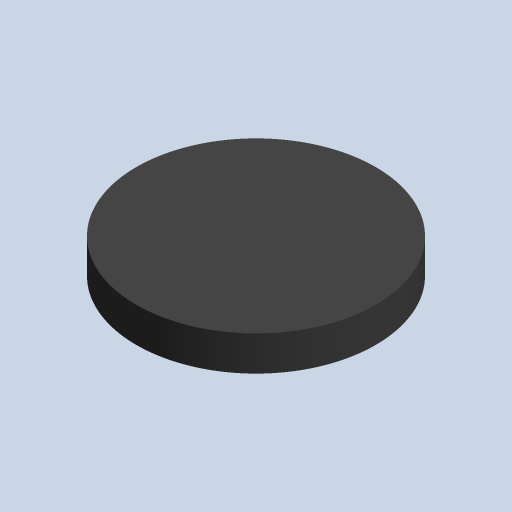
# Autodesk Inventor part: seal
Saved by Autodesk Inventor 2024 (Build 280153000, 153)
## iProperties
Part Number: seal
Material: Generic
Document SubType Name: Modeling
Designer: newic
Appearance: Default
Author: newic
Autodesk Inventor part; units mm, degrees
ref_plane "YZ Plane" through (0, 0, 0) normal (1, 0, 0) x (0, 1, 0)
ref_plane "XZ Plane" through (0, 0, 0) normal (0, 1, 0) x (-1, 0, 0)
ref_plane "XY Plane" through (0, 0, 0) normal (0, 0, 1) x (1, 0, 0)
sketch "Sketch1" plane through (0, 0, 0) normal (0, 1, 0) x (-1, 0, 0)
  line L0 (0, 0) -> (76.2002, 0) construction
  line L1 (76.2002, 0) -> (76.2002, -76.2002) construction
  line L2 (76.2002, -76.2002) -> (0, -76.2002) construction
  line L3 (0, -76.2002) -> (0, 0) construction
  circle A0 centre (38.1001, -38.1001) radius 21.8573
  circle A1 centre (38.1001, -38.1001) radius 20.8567
  line L4 (40.6618, -37.2458) -> (41.1876, -36.742)
  line L5 (41.1876, -36.742) -> (41.1876, -32.9593)
  spline S0 degree 4 poles (41.1876, -32.9593) (41.2926, -32.7172) (41.0043, -32.7956) (41.135, -32.4515) (40.8057, -32.605) knots 0 0 0 0 0 1 1 1 1 1
  line L6 (40.8057, -32.605) -> (40.0393, -32.605)
  arc A2 (40.0393, -31.6655) -> (40.0393, -32.605) centre (40.17, -32.1352) ccw
  line L7 (40.0393, -31.6655) -> (44.4894, -31.6655)
  arc A3 (44.4894, -32.605) -> (44.4894, -31.6655) centre (44.3665, -32.1352) ccw
  arc A4 (43.5252, -32.605) -> (43.1544, -32.9593) centre (43.4942, -32.9437) ccw
  line L8 (43.5252, -32.605) -> (44.4894, -32.605)
  line L9 (43.1544, -32.9593) -> (43.1544, -43.4953)
  line L10 (43.1544, -43.4953) -> (43.1877, -43.6584) construction
  line L11 (43.1877, -43.6584) -> (43.3031, -43.8163) construction
  line L12 (43.3031, -43.8163) -> (43.4033, -43.8706) construction
  line L13 (43.4033, -43.8706) -> (43.573, -43.9418) construction
  line L14 (43.573, -43.9418) -> (43.84, -44.0167) construction
  line L15 (43.84, -44.0167) -> (44.112, -44.0167) construction
  line L16 (44.112, -44.0167) -> (44.5627, -44.11) construction
  line L17 (44.5627, -44.11) -> (44.6715, -44.1722) construction
  line L18 (44.6715, -44.1722) -> (44.9163, -44.3198) construction
  line L19 (44.9163, -44.3198) -> (45.0154, -44.4232) construction
  line L20 (45.0154, -44.4232) -> (45.0834, -44.5452) construction
  line L21 (45.0834, -44.5452) -> (45.0834, -44.6618) construction
  line L22 (45.0834, -44.6618) -> (45.1145, -44.7939) construction
  line L23 (45.1145, -44.7939) -> (44.9878, -44.9153) construction
  line L24 (44.9878, -44.9153) -> (44.7842, -45.0076) construction
  line L25 (44.7842, -45.0076) -> (44.6482, -45.0076) construction
  spline S1 degree 4 poles (43.1544, -43.4953) (43.1877, -43.6584) (43.3031, -43.8163) (43.4033, -43.8706) (43.573, -43.9418) (43.84, -44.0167) (44.112, -44.0167) (44.5627, -44.11) (44.6715, -44.1722) (44.9163, -44.3198) (45.0154, -44.4232) (45.0834, -44.5452) (45.0834, -44.6618) (45.1145, -44.7939) (44.9878, -44.9153) (44.7842, -45.0076) (44.6482, -45.0076) knots 1 1 1 1 1 2 3 4 5 6 7 8 9 10 11 12 13 14 14 14 14 14
  arc A5 (44.6482, -45.0076) -> (39.9953, -45.0076) centre (42.3218, -57.2669) ccw
  line L26 (39.9953, -45.0076) -> (39.6196, -45.0402) construction
  line L27 (39.6196, -45.0402) -> (39.4833, -44.9615) construction
  line L28 (39.4833, -44.9615) -> (39.3855, -44.9153) construction
  line L29 (39.3855, -44.9153) -> (39.2941, -44.7888) construction
  line L30 (39.2941, -44.7888) -> (39.2941, -44.6035) construction
  line L31 (39.2941, -44.6035) -> (39.3481, -44.504) construction
  line L32 (39.3481, -44.504) -> (39.4207, -44.3715) construction
  line L33 (39.4207, -44.3715) -> (39.6288, -44.2164) construction
  line L34 (39.6288, -44.2164) -> (39.9032, -44.1411) construction
  line L35 (39.9032, -44.1411) -> (40.2033, -44.0797) construction
  line L36 (40.2033, -44.0797) -> (40.4675, -44.0634) construction
  line L37 (40.4675, -44.0634) -> (40.7103, -44.0167) construction
  line L38 (40.7103, -44.0167) -> (40.902, -43.9418) construction
  line L39 (40.902, -43.9418) -> (41.1242, -43.7775) construction
  line L40 (41.1242, -43.7775) -> (41.2453, -43.71) construction
  line L41 (41.2453, -43.71) -> (41.2975, -43.5237) construction
  spline S2 degree 4 poles (39.9953, -45.0076) (39.6196, -45.0402) (39.4833, -44.9615) (39.3855, -44.9153) (39.2941, -44.7888) (39.2941, -44.6035) (39.3481, -44.504) (39.4207, -44.3715) (39.6288, -44.2164) (39.9032, -44.1411) (40.2033, -44.0797) (40.4675, -44.0634) (40.7103, -44.0167) (40.902, -43.9418) (41.1242, -43.7775) (41.2453, -43.71) (41.2975, -43.5237) knots 1 1 1 1 1 2 3 4 5 6 7 8 9 10 11 12 13 14 14 14 14 14
  line L42 (41.2975, -43.5237) -> (41.2975, -40.0842)
  line L43 (41.2975, -40.0842) -> (40.7103, -39.4498)
  line L44 (40.7103, -39.4498) -> (34.7202, -39.4498)
  line L45 (40.6618, -37.2458) -> (34.7686, -37.2458)
  line L46 (34.7686, -37.2458) -> (34.2429, -36.742)
  line L47 (34.2429, -36.742) -> (34.2429, -32.9593)
  spline S3 degree 4 poles (34.2429, -32.9593) (34.1682, -32.7875) (34.3486, -32.6326) (34.3667, -32.6001) (34.6248, -32.605) knots 0 0 0 0 0 1 1 1 1 1
  line L48 (34.6248, -32.605) -> (35.3912, -32.605)
  arc A6 (35.3912, -32.605) -> (35.3912, -31.6655) centre (35.2605, -32.1352) ccw
  line L49 (35.3912, -31.6655) -> (30.941, -31.6655)
  arc A7 (30.941, -31.6655) -> (30.941, -32.605) centre (31.064, -32.1352) ccw
  arc A8 (32.2761, -32.9593) -> (31.9052, -32.605) centre (31.9363, -32.9437) ccw
  line L50 (31.9052, -32.605) -> (30.941, -32.605)
  line L51 (32.2761, -32.9593) -> (32.2761, -43.4953)
  line L52 (32.2761, -43.4953) -> (32.2427, -43.6584) construction
  line L53 (32.2427, -43.6584) -> (32.1273, -43.8163) construction
  line L54 (32.1273, -43.8163) -> (32.0272, -43.8706) construction
  line L55 (32.0272, -43.8706) -> (31.8575, -43.9418) construction
  line L56 (31.8575, -43.9418) -> (31.5905, -44.0167) construction
  line L57 (31.5905, -44.0167) -> (31.3185, -44.0167) construction
  line L58 (31.3185, -44.0167) -> (30.8677, -44.11) construction
  line L59 (30.8677, -44.11) -> (30.7589, -44.1722) construction
  line L60 (30.7589, -44.1722) -> (30.5141, -44.3198) construction
  line L61 (30.5141, -44.3198) -> (30.415, -44.4232) construction
  line L62 (30.415, -44.4232) -> (30.347, -44.5452) construction
  line L63 (30.347, -44.5452) -> (30.347, -44.6618) construction
  line L64 (30.347, -44.6618) -> (30.316, -44.7939) construction
  line L65 (30.316, -44.7939) -> (30.4426, -44.9153) construction
  line L66 (30.4426, -44.9153) -> (30.6462, -45.0076) construction
  line L67 (30.6462, -45.0076) -> (30.7822, -45.0076) construction
  spline S4 degree 4 poles (32.2761, -43.4953) (32.2427, -43.6584) (32.1273, -43.8163) (32.0272, -43.8706) (31.8575, -43.9418) (31.5905, -44.0167) (31.3185, -44.0167) (30.8677, -44.11) (30.7589, -44.1722) (30.5141, -44.3198) (30.415, -44.4232) (30.347, -44.5452) (30.347, -44.6618) (30.316, -44.7939) (30.4426, -44.9153) (30.6462, -45.0076) (30.7822, -45.0076) knots 1 1 1 1 1 2 3 4 5 6 7 8 9 10 11 12 13 14 14 14 14 14
  arc A9 (35.4351, -45.0076) -> (30.7822, -45.0076) centre (33.1087, -57.2669) ccw
  line L68 (35.4351, -45.0076) -> (35.8108, -45.0402) construction
  line L69 (35.8108, -45.0402) -> (35.9472, -44.9615) construction
  line L70 (35.9472, -44.9615) -> (36.0449, -44.9153) construction
  line L71 (36.0449, -44.9153) -> (36.1363, -44.7888) construction
  line L72 (36.1363, -44.7888) -> (36.1363, -44.6035) construction
  line L73 (36.1363, -44.6035) -> (36.0824, -44.504) construction
  line L74 (36.0824, -44.504) -> (36.0098, -44.3715) construction
  line L75 (36.0098, -44.3715) -> (35.8017, -44.2164) construction
  line L76 (35.8017, -44.2164) -> (35.5273, -44.1411) construction
  line L77 (35.5273, -44.1411) -> (35.2272, -44.0797) construction
  line L78 (35.2272, -44.0797) -> (34.963, -44.0634) construction
  line L79 (34.963, -44.0634) -> (34.7202, -44.0167) construction
  line L80 (34.7202, -44.0167) -> (34.5284, -43.9418) construction
  line L81 (34.5284, -43.9418) -> (34.3063, -43.7775) construction
  line L82 (34.3063, -43.7775) -> (34.1852, -43.71) construction
  line L83 (34.1852, -43.71) -> (34.1329, -43.5237) construction
  spline S5 degree 4 poles (35.4351, -45.0076) (35.8108, -45.0402) (35.9472, -44.9615) (36.0449, -44.9153) (36.1363, -44.7888) (36.1363, -44.6035) (36.0824, -44.504) (36.0098, -44.3715) (35.8017, -44.2164) (35.5273, -44.1411) (35.2272, -44.0797) (34.963, -44.0634) (34.7202, -44.0167) (34.5284, -43.9418) (34.3063, -43.7775) (34.1852, -43.71) (34.1329, -43.5237) knots 1 1 1 1 1 2 3 4 5 6 7 8 9 10 11 12 13 14 14 14 14 14
  line L84 (34.1329, -43.5237) -> (34.1329, -40.0842)
  line L85 (34.1329, -40.0842) -> (34.7202, -39.4498)
  line L86 (34.7202, -39.4498) -> (40.7103, -39.4498)
  line L87 (38.2912, -52.5831) -> (38.0672, -52.5831)
  line L88 (48.7025, -50.0158) -> (49.2279, -50.0158)
  line L89 (49.2279, -50.0158) -> (49.761, -50.4057)
  line L90 (49.761, -50.4057) -> (49.8872, -50.2845) construction
  line L91 (49.8872, -50.2845) -> (50.0462, -50.1321) construction
  line L92 (50.0462, -50.1321) -> (50.1401, -49.9591) construction
  line L93 (50.1401, -49.9591) -> (50.3738, -49.7351) construction
  line L94 (50.3738, -49.7351) -> (50.6671, -49.443) construction
  line L95 (50.6671, -49.443) -> (50.9264, -49.1944) construction
  line L96 (50.9264, -49.1944) -> (51.1372, -48.9924) construction
  line L97 (51.1372, -48.9924) -> (51.7205, -48.3816) construction
  line L98 (51.7205, -48.3816) -> (52.1066, -47.8535) construction
  line L99 (52.1066, -47.8535) -> (52.4867, -47.4569) construction
  line L100 (52.4867, -47.4569) -> (52.8214, -46.9579) construction
  line L101 (52.8214, -46.9579) -> (53.2913, -46.4144) construction
  line L102 (53.2913, -46.4144) -> (53.7244, -45.822) construction
  line L103 (53.7244, -45.822) -> (53.8819, -45.6067) construction
  line L104 (53.8819, -45.6067) -> (54.0234, -45.2698) construction
  line L105 (54.0234, -45.2698) -> (54.098, -45.1983) construction
  line L106 (54.098, -45.1983) -> (54.069, -45.1461) construction
  line L107 (54.069, -45.1461) -> (54.0322, -45.1077) construction
  line L108 (54.0322, -45.1077) -> (53.8711, -44.9534) construction
  line L109 (53.8711, -44.9534) -> (53.6017, -44.6962) construction
  line L110 (53.6017, -44.6962) -> (53.2876, -44.11) construction
  line L111 (53.2876, -44.11) -> (52.7307, -43.3484) construction
  line L112 (52.7307, -43.3484) -> (52.267, -42.5166) construction
  line L113 (52.267, -42.5166) -> (51.2177, -40.6344) construction
  line L114 (51.2177, -40.6344) -> (50.2882, -38.5878) construction
  line L115 (50.2882, -38.5878) -> (49.761, -37.085) construction
  line L116 (49.761, -37.085) -> (49.1388, -35.28) construction
  line L117 (49.1388, -35.28) -> (48.4341, -32.6978) construction
  line L118 (48.4341, -32.6978) -> (48.4341, -32.3678) construction
  line L119 (48.4341, -32.3678) -> (48.2809, -31.6655) construction
  line L120 (48.2809, -31.6655) -> (48.2661, -31.5479) construction
  spline S6 degree 4 poles (49.761, -50.4057) (49.8872, -50.2845) (50.0462, -50.1321) (50.1401, -49.9591) (50.3738, -49.7351) (50.6671, -49.443) (50.9264, -49.1944) (51.1372, -48.9924) (51.7205, -48.3816) (52.1066, -47.8535) (52.4867, -47.4569) (52.8214, -46.9579) (53.2913, -46.4144) (53.7244, -45.822) (53.8819, -45.6067) (54.0234, -45.2698) (54.098, -45.1983) (54.069, -45.1461) (54.0322, -45.1077) (53.8711, -44.9534) (53.6017, -44.6962) (53.2876, -44.11) (52.7307, -43.3484) (52.267, -42.5166) (51.2177, -40.6344) (50.2882, -38.5878) (49.761, -37.085) (49.1388, -35.28) (48.4341, -32.6978) (48.4341, -32.3678) (48.2809, -31.6655) (48.2661, -31.5479) knots 1 1 1 1 1 2 3 4 5 6 7 8 9 10 11 12 13 14 15 16 17 18 19 20 21 22 23 24 25 26 27 28 29 29 29 29 29
  line L121 (48.2661, -31.5479) -> (48.2274, -31.2403) construction
  line L122 (48.2274, -31.2403) -> (48.2541, -30.9327) construction
  line L123 (48.2541, -30.9327) -> (48.2541, -30.7642) construction
  line L124 (48.2541, -30.7642) -> (48.3417, -30.5558) construction
  line L125 (48.3417, -30.5558) -> (48.3952, -30.5045) construction
  line L126 (48.3952, -30.5045) -> (48.5589, -30.5384) construction
  line L127 (48.5589, -30.5384) -> (48.7025, -30.6473) construction
  line L128 (48.7025, -30.6473) -> (48.8728, -30.8478) construction
  line L129 (48.8728, -30.8478) -> (49.1688, -31.1565) construction
  line L130 (49.1688, -31.1565) -> (49.5553, -31.6852) construction
  line L131 (49.5553, -31.6852) -> (49.8872, -32.0507) construction
  line L132 (49.8872, -32.0507) -> (50.2882, -32.3413) construction
  line L133 (50.2882, -32.3413) -> (50.6084, -32.4076) construction
  line L134 (50.6084, -32.4076) -> (50.7152, -32.3052) construction
  line L135 (50.7152, -32.3052) -> (50.9957, -32.2478) construction
  line L136 (50.9957, -32.2478) -> (51.3083, -31.9482) construction
  line L137 (51.3083, -31.9482) -> (51.4714, -31.7252) construction
  line L138 (51.4714, -31.7252) -> (51.7423, -31.4649) construction
  line L139 (51.7423, -31.4649) -> (51.9587, -31.4195) construction
  line L140 (51.9587, -31.4195) -> (52.142, -31.2439) construction
  line L141 (52.142, -31.2439) -> (52.267, -31.1341) construction
  line L142 (52.267, -31.1341) -> (52.1937, -31.0543) construction
  line L143 (52.1937, -31.0543) -> (52.1066, -30.9669) construction
  line L144 (52.1066, -30.9669) -> (51.9585, -30.9254) construction
  line L145 (51.9585, -30.9254) -> (51.6761, -30.867) construction
  line L146 (51.6761, -30.867) -> (51.5091, -30.6926) construction
  line L147 (51.5091, -30.6926) -> (51.2639, -30.5134) construction
  line L148 (51.2639, -30.5134) -> (51.1401, -30.3836) construction
  line L149 (51.1401, -30.3836) -> (51.0087, -30.2039) construction
  line L150 (51.0087, -30.2039) -> (51.0087, -29.9872) construction
  line L151 (51.0087, -29.9872) -> (51.1613, -29.775) construction
  line L152 (51.1613, -29.775) -> (51.5939, -29.3746) construction
  line L153 (51.5939, -29.3746) -> (51.9135, -29.0787) construction
  line L154 (51.9135, -29.0787) -> (52.1836, -28.8286) construction
  line L155 (52.1836, -28.8286) -> (52.3342, -28.4702) construction
  line L156 (52.3342, -28.4702) -> (52.6833, -27.9927) construction
  line L157 (52.6833, -27.9927) -> (52.9107, -27.5734) construction
  line L158 (52.9107, -27.5734) -> (53.0092, -27.2183) construction
  line L159 (53.0092, -27.2183) -> (52.7307, -26.5536) construction
  line L160 (52.7307, -26.5536) -> (52.4989, -26.1497) construction
  line L161 (52.4989, -26.1497) -> (52.1641, -25.9049) construction
  line L162 (52.1641, -25.9049) -> (51.1372, -25.108) construction
  line L163 (51.1372, -25.108) -> (50.3531, -24.635) construction
  line L164 (50.3531, -24.635) -> (49.721, -24.211) construction
  line L165 (49.721, -24.211) -> (49.1894, -23.9238) construction
  line L166 (49.1894, -23.9238) -> (48.8873, -23.6086) construction
  line L167 (48.8873, -23.6086) -> (48.2185, -23.1196) construction
  line L168 (48.2185, -23.1196) -> (47.9551, -22.7594) construction
  line L169 (47.9551, -22.7594) -> (47.6777, -22.4563) construction
  line L170 (47.6777, -22.4563) -> (47.3154, -22.3042) construction
  line L171 (47.3154, -22.3042) -> (47.0473, -22.1916) construction
  line L172 (47.0473, -22.1916) -> (46.6874, -22.1916) construction
  line L173 (46.6874, -22.1916) -> (46.317, -22.2339) construction
  line L174 (46.317, -22.2339) -> (45.9234, -22.3551) construction
  line L175 (45.9234, -22.3551) -> (45.2614, -22.5181) construction
  line L176 (45.2614, -22.5181) -> (44.803, -22.7218) construction
  line L177 (44.803, -22.7218) -> (44.304, -22.9323) construction
  line L178 (44.304, -22.9323) -> (42.7641, -23.6271) construction
  spline S7 degree 4 poles (48.2661, -31.5479) (48.2274, -31.2403) (48.2541, -30.9327) (48.2541, -30.7642) (48.3417, -30.5558) (48.3952, -30.5045) (48.5589, -30.5384) (48.7025, -30.6473) (48.8728, -30.8478) (49.1688, -31.1565) (49.5553, -31.6852) (49.8872, -32.0507) (50.2882, -32.3413) (50.6084, -32.4076) (50.7152, -32.3052) (50.9957, -32.2478) (51.3083, -31.9482) (51.4714, -31.7252) (51.7423, -31.4649) (51.9587, -31.4195) (52.142, -31.2439) (52.267, -31.1341) (52.1937, -31.0543) (52.1066, -30.9669) (51.9585, -30.9254) (51.6761, -30.867) (51.5091, -30.6926) (51.2639, -30.5134) (51.1401, -30.3836) (51.0087, -30.2039) (51.0087, -29.9872) (51.1613, -29.775) (51.5939, -29.3746) (51.9135, -29.0787) (52.1836, -28.8286) (52.3342, -28.4702) (52.6833, -27.9927) (52.9107, -27.5734) (53.0092, -27.2183) (52.7307, -26.5536) (52.4989, -26.1497) (52.1641, -25.9049) (51.1372, -25.108) (50.3531, -24.635) (49.721, -24.211) (49.1894, -23.9238) (48.8873, -23.6086) (48.2185, -23.1196) (47.9551, -22.7594) (47.6777, -22.4563) (47.3154, -22.3042) (47.0473, -22.1916) (46.6874, -22.1916) (46.317, -22.2339) (45.9234, -22.3551) (45.2614, -22.5181) (44.803, -22.7218) (44.304, -22.9323) (42.7641, -23.6271) (42.1419, -23.8519) (41.7933, -23.9841) (41.6423, -24.0391) knots 1 1 1 1 1 2 3 4 5 6 7 8 9 10 11 12 13 14 15 16 17 18 19 20 21 22 23 24 25 26 27 28 29 30 31 32 33 34 35 36 37 38 39 40 41 42 43 44 45 46 47 48 49 50 51 52 53 54 55 56 57 58 58.816263 58.816263 58.816263 58.816263 58.816263
  line L179 (39.2968, -24.3991) -> (40.7554, -24.3991)
  line L180 (40.7554, -24.3991) -> (41.6423, -24.0391)
  line L181 (42.7641, -23.6271) -> (42.1419, -23.8519) construction
  line L182 (42.1419, -23.8519) -> (41.7933, -23.9841) construction
  line L183 (41.7933, -23.9841) -> (41.6423, -24.0391) construction
  line L184 (39.2968, -24.3991) -> (39.2433, -24.4111) construction
  line L185 (39.2433, -24.4111) -> (39.1663, -24.4723) construction
  line L186 (39.1663, -24.4723) -> (39.1175, -24.5601) construction
  line L187 (39.1175, -24.5601) -> (39.0699, -24.7134) construction
  line L188 (39.0699, -24.7134) -> (39.0012, -25.0007) construction
  line L189 (39.0012, -25.0007) -> (38.7576, -25.3192) construction
  line L190 (38.7576, -25.3192) -> (38.4704, -25.6314) construction
  line L191 (38.4704, -25.6314) -> (38.1769, -25.9186) construction
  line L192 (38.1769, -25.9186) -> (38.0838, -25.973) construction
  spline S8 degree 4 poles (39.2968, -24.3991) (39.2433, -24.4111) (39.1663, -24.4723) (39.1175, -24.5601) (39.0699, -24.7134) (39.0012, -25.0007) (38.7576, -25.3192) (38.4704, -25.6314) (38.1769, -25.9186) (38.0838, -25.973) knots 1 1 1 1 1 2 3 4 5 6 7 7 7 7 7
  line L193 (38.0838, -25.973) -> (37.6286, -25.973)
  line L194 (37.8562, -25.973) -> (38.1001, -56.7349)
  arc A10 (38.1001, -56.7349) -> (38.5091, -56.4718) centre (38.0456, -56.2007) ccw
  arc A11 (38.6312, -56.0666) -> (38.5091, -56.4718) centre (39.5479, -56.5638) ccw
  arc A12 (39.0699, -55.3511) -> (38.6312, -56.0666) centre (40.3438, -56.6243) ccw
  arc A13 (39.7556, -54.7188) -> (39.0699, -55.3511) centre (41.8297, -57.6563) ccw
  arc A14 (43.3532, -53.0725) -> (39.7556, -54.7188) centre (46.6536, -65.0391) ccw
  arc A15 (43.3532, -53.0725) -> (46.2754, -51.8022) centre (38.528, -37.9773) ccw
  arc A16 (46.2754, -51.8022) -> (48.7025, -50.0158) centre (44.0006, -46.1692) ccw
  line L195 (27.3925, -50.1848) -> (26.8671, -50.1931)
  line L196 (26.8671, -50.1931) -> (26.3403, -50.5913)
  line L197 (26.3403, -50.5913) -> (26.2121, -50.4722) construction
  line L198 (26.2121, -50.4722) -> (26.0508, -50.3224) construction
  line L199 (26.0508, -50.3224) -> (25.9542, -50.1509) construction
  line L200 (25.9542, -50.1509) -> (25.7169, -49.9306) construction
  line L201 (25.7169, -49.9306) -> (25.4191, -49.6431) construction
  line L202 (25.4191, -49.6431) -> (25.1558, -49.3987) construction
  line L203 (25.1558, -49.3987) -> (24.9419, -49.2001) construction
  line L204 (24.9419, -49.2001) -> (24.349, -48.5986) construction
  line L205 (24.349, -48.5986) -> (23.9545, -48.0767) construction
  line L206 (23.9545, -48.0767) -> (23.5682, -47.6861) construction
  line L207 (23.5682, -47.6861) -> (23.2255, -47.1925) construction
  line L208 (23.2255, -47.1925) -> (22.7471, -46.6565) construction
  line L209 (22.7471, -46.6565) -> (22.3047, -46.0711) construction
  line L210 (22.3047, -46.0711) -> (22.1438, -45.8583) construction
  line L211 (22.1438, -45.8583) -> (21.997, -45.5237) construction
  line L212 (21.997, -45.5237) -> (21.9212, -45.4533) construction
  line L213 (21.9212, -45.4533) -> (21.9495, -45.4007) construction
  line L214 (21.9495, -45.4007) -> (21.9857, -45.3618) construction
  line L215 (21.9857, -45.3618) -> (22.1442, -45.2049) construction
  line L216 (22.1442, -45.2049) -> (22.4095, -44.9434) construction
  line L217 (22.4095, -44.9434) -> (22.7143, -44.3524) construction
  line L218 (22.7143, -44.3524) -> (23.259, -43.5821) construction
  line L219 (23.259, -43.5821) -> (23.7095, -42.743) construction
  line L220 (23.7095, -42.743) -> (24.7289, -40.8444) construction
  line L221 (24.7289, -40.8444) -> (25.6258, -38.7833) construction
  line L222 (25.6258, -38.7833) -> (26.1291, -37.2724) construction
  line L223 (26.1291, -37.2724) -> (26.7226, -35.4578) construction
  line L224 (26.7226, -35.4578) -> (27.3863, -32.8646) construction
  line L225 (27.3863, -32.8646) -> (27.381, -32.5347) construction
  line L226 (27.381, -32.5347) -> (27.5231, -31.8301) construction
  line L227 (27.5231, -31.8301) -> (27.536, -31.7122) construction
  spline S9 degree 4 poles (26.3403, -50.5913) (26.2121, -50.4722) (26.0508, -50.3224) (25.9542, -50.1509) (25.7169, -49.9306) (25.4191, -49.6431) (25.1558, -49.3987) (24.9419, -49.2001) (24.349, -48.5986) (23.9545, -48.0767) (23.5682, -47.6861) (23.2255, -47.1925) (22.7471, -46.6565) (22.3047, -46.0711) (22.1438, -45.8583) (21.997, -45.5237) (21.9212, -45.4533) (21.9495, -45.4007) (21.9857, -45.3618) (22.1442, -45.2049) (22.4095, -44.9434) (22.7143, -44.3524) (23.259, -43.5821) (23.7095, -42.743) (24.7289, -40.8444) (25.6258, -38.7833) (26.1291, -37.2724) (26.7226, -35.4578) (27.3863, -32.8646) (27.381, -32.5347) (27.5231, -31.8301) (27.536, -31.7122) knots 1 1 1 1 1 2 3 4 5 6 7 8 9 10 11 12 13 14 15 16 17 18 19 20 21 22 23 24 25 26 27 28 29 29 29 29 29
  line L228 (27.536, -31.7122) -> (27.5698, -31.4041) construction
  line L229 (27.5698, -31.4041) -> (27.5382, -31.0969) construction
  line L230 (27.5382, -31.0969) -> (27.5355, -30.9284) construction
  line L231 (27.5355, -30.9284) -> (27.4447, -30.7215) construction
  line L232 (27.4447, -30.7215) -> (27.3904, -30.671) construction
  line L233 (27.3904, -30.671) -> (27.2272, -30.7075) construction
  line L234 (27.2272, -30.7075) -> (27.0854, -30.8187) construction
  line L235 (27.0854, -30.8187) -> (26.9182, -31.0218) construction
  line L236 (26.9182, -31.0218) -> (26.6273, -31.3353) construction
  line L237 (26.6273, -31.3353) -> (26.2492, -31.8699) construction
  line L238 (26.2492, -31.8699) -> (25.9231, -32.2407) construction
  line L239 (25.9231, -32.2407) -> (25.5267, -32.5376) construction
  line L240 (25.5267, -32.5376) -> (25.2077, -32.609) construction
  line L241 (25.2077, -32.609) -> (25.0992, -32.5083) construction
  line L242 (25.0992, -32.5083) -> (24.8179, -32.4553) construction
  line L243 (24.8179, -32.4553) -> (24.5005, -32.1607) construction
  line L244 (24.5005, -32.1607) -> (24.3339, -31.9403) construction
  line L245 (24.3339, -31.9403) -> (24.0589, -31.6844) construction
  line L246 (24.0589, -31.6844) -> (23.8418, -31.6424) construction
  line L247 (23.8418, -31.6424) -> (23.6558, -31.4698) construction
  line L248 (23.6558, -31.4698) -> (23.529, -31.3619) construction
  line L249 (23.529, -31.3619) -> (23.6011, -31.281) construction
  line L250 (23.6011, -31.281) -> (23.6868, -31.1922) construction
  line L251 (23.6868, -31.1922) -> (23.8342, -31.1484) construction
  line L252 (23.8342, -31.1484) -> (24.1156, -31.0855) construction
  line L253 (24.1156, -31.0855) -> (24.2799, -30.9085) construction
  line L254 (24.2799, -30.9085) -> (24.5221, -30.7254) construction
  line L255 (24.5221, -30.7254) -> (24.6439, -30.5937) construction
  line L256 (24.6439, -30.5937) -> (24.7724, -30.4119) construction
  line L257 (24.7724, -30.4119) -> (24.769, -30.1953) construction
  line L258 (24.769, -30.1953) -> (24.6131, -29.9855) construction
  line L259 (24.6131, -29.9855) -> (24.1742, -29.5919) construction
  line L260 (24.1742, -29.5919) -> (23.8499, -29.3012) construction
  line L261 (23.8499, -29.3012) -> (23.5758, -29.0554) construction
  line L262 (23.5758, -29.0554) -> (23.4196, -28.6995) construction
  line L263 (23.4196, -28.6995) -> (23.0629, -28.2275) construction
  line L264 (23.0629, -28.2275) -> (22.8289, -27.8119) construction
  line L265 (22.8289, -27.8119) -> (22.7249, -27.4584) construction
  line L266 (22.7249, -27.4584) -> (22.9927, -26.7893) construction
  line L267 (22.9927, -26.7893) -> (23.2182, -26.3818) construction
  line L268 (23.2182, -26.3818) -> (23.549, -26.1318) construction
  line L269 (23.549, -26.1318) -> (24.5632, -25.3187) construction
  line L270 (24.5632, -25.3187) -> (25.3397, -24.8333) construction
  line L271 (25.3397, -24.8333) -> (25.9649, -24.3993) construction
  line L272 (25.9649, -24.3993) -> (26.492, -24.1038) construction
  line L273 (26.492, -24.1038) -> (26.789, -23.7838) construction
  line L274 (26.789, -23.7838) -> (27.45, -23.2843) construction
  line L275 (27.45, -23.2843) -> (27.7076, -22.9199) construction
  line L276 (27.7076, -22.9199) -> (27.9802, -22.6125) construction
  line L277 (27.9802, -22.6125) -> (28.34, -22.4546) construction
  line L278 (28.34, -22.4546) -> (28.6063, -22.3378) construction
  line L279 (28.6063, -22.3378) -> (28.9662, -22.3321) construction
  line L280 (28.9662, -22.3321) -> (29.3372, -22.3686) construction
  line L281 (29.3372, -22.3686) -> (29.7326, -22.4834) construction
  line L282 (29.7326, -22.4834) -> (30.3972, -22.6359) construction
  line L283 (30.3972, -22.6359) -> (30.8587, -22.8323) construction
  line L284 (30.8587, -22.8323) -> (31.361, -23.0349) construction
  line L285 (31.361, -23.0349) -> (32.9117, -23.7052) construction
  spline S10 degree 4 poles (27.536, -31.7122) (27.5698, -31.4041) (27.5382, -31.0969) (27.5355, -30.9284) (27.4447, -30.7215) (27.3904, -30.671) (27.2272, -30.7075) (27.0854, -30.8187) (26.9182, -31.0218) (26.6273, -31.3353) (26.2492, -31.8699) (25.9231, -32.2407) (25.5267, -32.5376) (25.2077, -32.609) (25.0992, -32.5083) (24.8179, -32.4553) (24.5005, -32.1607) (24.3339, -31.9403) (24.0589, -31.6844) (23.8418, -31.6424) (23.6558, -31.4698) (23.529, -31.3619) (23.6011, -31.281) (23.6868, -31.1922) (23.8342, -31.1484) (24.1156, -31.0855) (24.2799, -30.9085) (24.5221, -30.7254) (24.6439, -30.5937) (24.7724, -30.4119) (24.769, -30.1953) (24.6131, -29.9855) (24.1742, -29.5919) (23.8499, -29.3012) (23.5758, -29.0554) (23.4196, -28.6995) (23.0629, -28.2275) (22.8289, -27.8119) (22.7249, -27.4584) (22.9927, -26.7893) (23.2182, -26.3818) (23.549, -26.1318) (24.5632, -25.3187) (25.3397, -24.8333) (25.9649, -24.3993) (26.492, -24.1038) (26.789, -23.7838) (27.45, -23.2843) (27.7076, -22.9199) (27.9802, -22.6125) (28.34, -22.4546) (28.6063, -22.3378) (28.9662, -22.3321) (29.3372, -22.3686) (29.7326, -22.4834) (30.3972, -22.6359) (30.8587, -22.8323) (31.361, -23.0349) (32.9117, -23.7052) (33.5374, -23.9201) (33.8881, -24.0468) (34.0399, -24.0993) knots 1 1 1 1 1 2 3 4 5 6 7 8 9 10 11 12 13 14 15 16 17 18 19 20 21 22 23 24 25 26 27 28 29 30 31 32 33 34 35 36 37 38 39 40 41 42 43 44 45 46 47 48 49 50 51 52 53 54 55 56 57 58 58.816263 58.816263 58.816263 58.816263 58.816263
  line L286 (36.3908, -24.4221) -> (34.9324, -24.4452)
  line L287 (34.9324, -24.4452) -> (34.0399, -24.0993)
  line L288 (32.9117, -23.7052) -> (33.5374, -23.9201) construction
  line L289 (33.5374, -23.9201) -> (33.8881, -24.0468) construction
  line L290 (33.8881, -24.0468) -> (34.0399, -24.0993) construction
  line L291 (36.3908, -24.4221) -> (36.4445, -24.4333) construction
  line L292 (36.4445, -24.4333) -> (36.5225, -24.4932) construction
  line L293 (36.5225, -24.4932) -> (36.5727, -24.5802) construction
  line L294 (36.5727, -24.5802) -> (36.6227, -24.7328) construction
  line L295 (36.6227, -24.7328) -> (36.696, -25.019) construction
  line L296 (36.696, -25.019) -> (36.9445, -25.3335) construction
  line L297 (36.9445, -25.3335) -> (37.2367, -25.6412) construction
  line L298 (37.2367, -25.6412) -> (37.5347, -25.9237) construction
  line L299 (37.5347, -25.9237) -> (37.6287, -25.9766) construction
  spline S11 degree 4 poles (36.3908, -24.4221) (36.4445, -24.4333) (36.5225, -24.4932) (36.5727, -24.5802) (36.6227, -24.7328) (36.696, -25.019) (36.9445, -25.3335) (37.2367, -25.6412) (37.5347, -25.9237) (37.6287, -25.9766) knots 1 1 1 1 1 2 3 4 5 6 7 7 7 7 7
  line L300 (37.6287, -25.9766) -> (38.0837, -25.9694)
  arc A17 (29.8476, -51.9324) -> (32.7895, -53.1563) centre (37.3749, -37.9864) ccw
  arc A18 (27.3925, -50.1848) -> (29.8476, -51.9324) centre (32.0328, -46.2641) ccw
  arc A19 (36.1363, -54.4971) -> (32.7895, -53.1563) centre (28.5329, -68.6286) ccw
  arc A20 (37.5347, -55.923) -> (36.1363, -54.4971) centre (32.3957, -59.564) ccw
  arc A21 (37.5347, -55.923) -> (38.1001, -56.7349) centre (38.3931, -55.928) ccw
  line L301 (37.8765, -28.5293) -> (38.9353, -28.5293)
  spline S12 degree 4 poles (38.9353, -28.5293) (39.0734, -28.5153) (39.235, -28.4247) (39.7119, -27.9172) (40.0591, -27.4924) (40.3856, -27.2204) (40.628, -27.0204) (40.8114, -26.9226) (41.1862, -26.9437) (41.513, -26.9433) (41.6075, -26.8718) (42.1054, -26.7692) (42.4444, -26.5333) (42.9513, -26.4281) (43.3962, -26.1436) (43.8872, -26.1192) (44.318, -25.8883) (44.9007, -25.4806) (45.5398, -25.3135) (45.9229, -25.2078) (45.976, -25.0775) knots 0 0 0 0 0 0.112458 0.166879 0.220388 0.267174 0.311957 0.35453 0.394382 0.437668 0.482725 0.531671 0.587405 0.64421 0.700743 0.757907 0.816633 0.875573 1 1 1 1 1
  spline S13 degree 4 poles (45.976, -25.0775) (46.0524, -25.0518) (46.2811, -25.1254) (46.3903, -24.9958) (46.6702, -25.2353) (47.0934, -25.6298) (47.464, -26.0099) (48.1375, -26.4473) (48.7069, -26.8363) (48.9769, -27.0113) (49.2133, -27.1257) (49.3419, -27.2815) (49.4167, -27.3513) (49.417, -27.4775) (49.4428, -27.5915) (49.4153, -27.6867) (49.4243, -27.763) (49.3797, -27.8219) (49.2973, -27.8628) (49.0519, -27.8753) (48.2998, -27.8481) (47.8569, -27.8921) (47.342, -27.8307) (47.2381, -27.8825) knots 0 0 0 0 0 0.086112 0.127188 0.177084 0.240639 0.312756 0.380982 0.442012 0.491183 0.529078 0.56225 0.592572 0.620822 0.648025 0.672897 0.695594 0.720273 0.755564 0.802899 0.860568 1 1 1 1 1
  spline S14 degree 4 poles (47.2381, -27.8825) (46.8036, -28.0259) (47.051, -28.1864) (46.1354, -28.667) (46.0566, -28.9624) (45.8039, -29.1649) (45.7683, -29.3826) (45.7291, -29.5505) (45.7372, -29.905) (45.7435, -30.39) (45.7233, -31.2372) (45.7599, -31.4923) (45.7639, -32.3084) (45.8743, -32.614) knots 0 0 0 0 0 0.200798 0.275055 0.342735 0.398857 0.456316 0.520713 0.595619 0.677623 0.766008 1 1 1 1 1
  spline S15 degree 4 poles (45.8743, -32.614) (45.7137, -32.7724) (46.4665, -35.208) (46.2054, -35.0081) (47.0977, -38.1106) (47.4234, -38.399) (47.7686, -39.905) (48.3464, -40.926) (48.9437, -42.1085) (49.649, -43.4282) (49.9606, -43.8863) (50.2945, -44.3908) (50.4181, -44.6802) (50.5672, -44.9184) (50.7241, -45.0451) (50.6523, -45.271) (50.7075, -45.4133) (50.6412, -45.6406) (50.5067, -45.6223) (50.1523, -46.1961) (49.9325, -46.3664) (49.7247, -46.8301) (49.4855, -46.939) (49.2978, -47.2293) (49.1062, -47.4299) (48.6959, -47.4202) (48.1844, -47.3814) (47.7859, -47.4146) (47.7237, -47.4124) knots 0 0 0 0 0 0.134375 0.188708 0.241348 0.29581 0.348426 0.40505 0.457878 0.505294 0.54432 0.575023 0.601347 0.624473 0.645729 0.66569 0.684809 0.707628 0.733814 0.763178 0.794671 0.823839 0.850795 0.876094 0.903339 0.932407 1 1 1 1 1
  spline S16 degree 4 poles (47.7237, -47.4124) (47.6689, -47.3552) (47.1019, -47.8924) (47.0089, -48.1366) (46.4951, -48.4489) (46.089, -48.829) (45.6562, -48.9821) (44.5447, -49.6219) (43.7859, -50.0266) (42.4528, -50.6041) (41.6151, -50.7219) (41.3619, -50.8814) (40.6146, -51.2115) (40.1168, -51.4616) (39.6343, -51.7112) (39.4366, -51.694) (38.5975, -52.2427) (38.4596, -52.512) (38.2912, -52.5831) knots 0 0 0 0 0 0.113764 0.163279 0.21106 0.267998 0.333934 0.40973 0.487636 0.556975 0.621613 0.678854 0.732776 0.783921 0.833088 0.881666 1 1 1 1 1
  arc A22 (45.7691, -31.9153) -> (45.8743, -33.0106) centre (53.8311, -31.6934) ccw
  line L302 (37.8432, -52.5867) -> (38.0672, -52.5831)
  line L303 (37.8765, -28.5293) -> (36.8177, -28.546)
  spline S17 degree 4 poles (36.8177, -28.546) (36.6795, -28.5343) (36.5165, -28.4463) (36.0316, -27.9464) (35.6777, -27.5271) (35.3469, -27.2603) (35.1014, -27.0642) (34.9165, -26.9693) (34.542, -26.9964) (34.2153, -27.0011) (34.1196, -26.9312) (33.6202, -26.8364) (33.2775, -26.606) (32.7689, -26.5089) (32.3196, -26.2314) (31.8283, -26.2148) (31.3938, -25.9908) (30.8048, -25.5924) (30.1631, -25.4354) (29.7784, -25.3358) (29.7232, -25.2063) knots 0 0 0 0 0 0.112458 0.166879 0.220388 0.267174 0.311957 0.35453 0.394382 0.437668 0.482725 0.531671 0.587405 0.64421 0.700743 0.757907 0.816633 0.875573 1 1 1 1 1
  spline S18 degree 4 poles (29.7232, -25.2063) (29.6465, -25.1819) (29.4189, -25.2591) (29.3077, -25.1312) (29.0316, -25.3751) (28.6147, -25.7763) (28.2502, -26.1622) (27.5837, -26.6103) (27.0205, -27.0082) (26.7533, -27.1875) (26.5188, -27.3057) (26.3927, -27.4635) (26.319, -27.5345) (26.3207, -27.6606) (26.2967, -27.775) (26.3257, -27.8698) (26.3179, -27.9462) (26.3635, -28.0044) (26.4465, -28.044) (26.6921, -28.0526) (27.4436, -28.0134) (27.8872, -28.0504) (28.401, -27.9809) (28.5058, -28.031) knots 0 0 0 0 0 0.086112 0.127188 0.177084 0.240639 0.312756 0.380982 0.442012 0.491183 0.529078 0.56225 0.592572 0.620822 0.648025 0.672897 0.695594 0.720273 0.755564 0.802899 0.860568 1 1 1 1 1
  spline S19 degree 4 poles (28.5058, -28.031) (28.9425, -28.1675) (28.6976, -28.3319) (29.6208, -28.7979) (29.7042, -29.092) (29.9601, -29.2905) (29.9991, -29.5076) (30.041, -29.6749) (30.0385, -30.0295) (30.0399, -30.5145) (30.0736, -31.3613) (30.041, -31.6169) (30.05, -32.433) (29.9444, -32.7403) knots 0 0 0 0 0 0.200798 0.275055 0.342735 0.398857 0.456316 0.520713 0.595619 0.677623 0.766008 1 1 1 1 1
  spline S20 degree 4 poles (29.9444, -32.7403) (30.1074, -32.8962) (29.3934, -35.3434) (29.6513, -35.1393) (28.8083, -38.2556) (28.4872, -38.5492) (28.1659, -40.0604) (27.6044, -41.0905) (27.0259, -42.2822) (26.3416, -43.6129) (26.0373, -44.0759) (25.7115, -44.5857) (25.5925, -44.877) (25.4472, -45.1175) (25.2923, -45.2468) (25.3677, -45.4715) (25.3147, -45.6146) (25.3846, -45.8408) (25.5188, -45.8204) (25.8822, -46.3885) (26.1048, -46.5553) (26.3199, -47.0157) (26.5608, -47.1208) (26.753, -47.408) (26.9478, -47.6055) (27.3579, -47.5894) (27.8688, -47.5424) (28.2677, -47.5694) (28.3298, -47.5661) knots 0 0 0 0 0 0.134375 0.188708 0.241348 0.29581 0.348426 0.40505 0.457878 0.505294 0.54432 0.575023 0.601347 0.624473 0.645729 0.66569 0.684809 0.707628 0.733814 0.763178 0.794671 0.823839 0.850795 0.876094 0.903339 0.932407 1 1 1 1 1
  spline S21 degree 4 poles (28.3298, -47.5661) (28.3837, -47.5081) (28.9592, -48.0362) (29.0561, -48.2789) (29.5748, -48.583) (29.9868, -48.9567) (30.422, -49.1029) (31.5435, -49.7249) (32.3087, -50.1176) (33.6507, -50.6739) (34.4901, -50.7784) (34.7459, -50.9338) (35.4983, -51.2521) (36, -51.4942) (36.4864, -51.7362) (36.6838, -51.7158) (37.5315, -52.2512) (37.6737, -52.5182) (37.8432, -52.5867) knots 0 0 0 0 0 0.113764 0.163279 0.21106 0.267998 0.333934 0.40973 0.487636 0.556975 0.621613 0.678854 0.732776 0.783921 0.833088 0.881666 1 1 1 1 1
  arc A23 (29.9507, -33.1368) -> (30.0385, -32.04) centre (21.9741, -31.9459) ccw
  point P0 (41.1876, -32.7945)
  point P1 (41.1175, -32.7003)
  point P2 (41.0347, -32.6044)
  point P3 (34.2429, -32.7945)
  point P4 (34.3146, -32.6857)
  point P5 (34.4094, -32.6264)
  point P6 (37.8764, -52.5831)
  point P7 (39.089, -28.4833)
  point P8 (39.3429, -28.288)
  point P9 (39.7723, -27.8334)
  point P10 (40.1126, -27.4629)
  point P11 (40.4198, -27.1929)
  point P12 (40.6354, -27.0288)
  point P13 (40.8285, -26.9501)
  point P14 (41.2, -26.94)
  point P15 (41.4803, -26.9267)
  point P16 (41.6228, -26.8853)
  point P17 (41.9993, -26.7707)
  point P18 (42.4444, -26.5736)
  point P19 (42.9352, -26.3938)
  point P20 (43.4169, -26.1915)
  point P21 (43.8665, -26.0803)
  point P22 (44.2933, -25.888)
  point P23 (44.784, -25.5999)
  point P24 (45.3799, -25.3642)
  point P25 (45.8296, -25.2031)
  point P26 (46.1504, -25.0771)
  point P27 (46.3165, -25.0767)
  point P28 (46.4224, -25.0764)
  point P29 (46.5835, -25.1668)
  point P30 (46.9803, -25.5281)
  point P31 (47.4705, -25.9756)
  point P32 (48.2156, -26.5036)
  point P33 (48.7811, -26.882)
  point P34 (49.0427, -27.0404)
  point P35 (49.2365, -27.1696)
  point P36 (49.3528, -27.2892)
  point P37 (49.4034, -27.3669)
  point P38 (49.4222, -27.4776)
  point P39 (49.4318, -27.6005)
  point P40 (49.421, -27.6978)
  point P41 (49.4133, -27.763)
  point P42 (49.3857, -27.8068)
  point P43 (49.3323, -27.84)
  point P44 (49.1709, -27.8656)
  point P45 (48.6145, -27.8643)
  point P46 (48.001, -27.8673)
  point P47 (47.4717, -27.8578)
  point P48 (46.8894, -28.1129)
  point P49 (46.6026, -28.4088)
  point P50 (46.1438, -28.7961)
  point P51 (45.9922, -28.994)
  point P52 (45.828, -29.196)
  point P53 (45.7691, -29.3686)
  point P54 (45.7438, -29.5243)
  point P55 (45.7354, -29.819)
  point P56 (45.7396, -30.362)
  point P57 (45.7354, -30.9555)
  point P58 (45.7438, -31.3512)
  point P59 (45.7691, -31.9153)
  point P60 (45.9942, -33.6055)
  point P61 (46.3327, -35.0802)
  point P62 (46.5362, -36.0535)
  point P63 (47.1136, -37.9207)
  point P64 (47.4085, -38.5892)
  point P65 (47.7829, -39.718)
  point P66 (48.3291, -40.9156)
  point P67 (49.0472, -42.2916)
  point P68 (49.7271, -43.5211)
  point P69 (50.0539, -44.0296)
  point P70 (50.3093, -44.4497)
  point P71 (50.4512, -44.7218)
  point P72 (50.5932, -44.9263)
  point P73 (50.681, -45.0759)
  point P74 (50.6761, -45.2671)
  point P75 (50.6841, -45.4268)
  point P76 (50.6413, -45.5746)
  point P77 (50.5521, -45.6554)
  point P78 (50.2038, -46.0828)
  point P79 (49.9222, -46.4452)
  point P80 (49.6831, -46.8003)
  point P81 (49.4832, -46.9862)
  point P82 (49.29, -47.22)
  point P83 (49.1034, -47.3791)
  point P84 (48.8385, -47.4196)
  point P85 (48.3724, -47.4025)
  point P86 (47.881, -47.4072)
  point P87 (47.5036, -47.5404)
  point P88 (47.0699, -47.983)
  point P89 (46.848, -48.2092)
  point P90 (46.5345, -48.4436)
  point P91 (46.1544, -48.737)
  point P92 (45.7343, -48.9718)
  point P93 (44.7507, -49.4991)
  point P94 (43.6554, -50.0665)
  point P95 (42.2542, -50.5993)
  point P96 (41.6228, -50.7621)
  point P97 (41.2973, -50.9002)
  point P98 (40.6313, -51.211)
  point P99 (40.0196, -51.5119)
  point P100 (39.6595, -51.6747)
  point P101 (39.4722, -51.7388)
  point P102 (38.9838, -52.0199)
  point P103 (38.5003, -52.4245)
  point P104 (38.2579, -52.5801)
  point P105 (36.6633, -28.5026)
  point P106 (36.4064, -28.3113)
  point P107 (35.9698, -27.8635)
  point P108 (35.6237, -27.4985)
  point P109 (35.3123, -27.2334)
  point P110 (35.0941, -27.0727)
  point P111 (34.8998, -26.9971)
  point P112 (34.5281, -26.9929)
  point P113 (34.2477, -26.9841)
  point P114 (34.1045, -26.9449)
  point P115 (33.7263, -26.8363)
  point P116 (33.2781, -26.6463)
  point P117 (32.7845, -26.4743)
  point P118 (32.2997, -26.2796)
  point P119 (31.8484, -26.1755)
  point P120 (31.4185, -25.9901)
  point P121 (30.9233, -25.7098)
  point P122 (30.3238, -25.4836)
  point P123 (29.8716, -25.3296)
  point P124 (29.5489, -25.2087)
  point P125 (29.3827, -25.211)
  point P126 (29.2768, -25.2123)
  point P127 (29.1173, -25.3052)
  point P128 (28.7262, -25.6728)
  point P129 (28.2432, -26.128)
  point P130 (27.5065, -26.6677)
  point P131 (26.9471, -27.0551)
  point P132 (26.688, -27.2176)
  point P133 (26.4963, -27.3499)
  point P134 (26.3819, -27.4713)
  point P135 (26.3325, -27.5498)
  point P136 (26.3156, -27.6608)
  point P137 (26.3079, -27.7839)
  point P138 (26.3202, -27.8809)
  point P139 (26.3289, -27.946)
  point P140 (26.3572, -27.9894)
  point P141 (26.4111, -28.0217)
  point P142 (26.573, -28.0448)
  point P143 (27.1293, -28.0346)
  point P144 (27.7427, -28.0279)
  point P145 (28.2718, -28.01)
  point P146 (28.8581, -28.2559)
  point P147 (29.1496, -28.5472)
  point P148 (29.6145, -28.9272)
  point P149 (29.7691, -29.1226)
  point P150 (29.9365, -29.322)
  point P151 (29.9981, -29.4936)
  point P152 (30.0259, -29.6489)
  point P153 (30.039, -29.9434)
  point P154 (30.0434, -30.4864)
  point P155 (30.057, -31.0798)
  point P156 (30.0548, -31.4756)
  point P157 (30.0385, -32.04)
  point P158 (29.8402, -33.7336)
  point P159 (29.5251, -35.2135)
  point P160 (29.3371, -36.1898)
  point P161 (28.7894, -38.066)
  point P162 (28.5051, -38.7391)
  point P163 (28.1487, -39.8736)
  point P164 (27.6215, -41.0798)
  point P165 (26.9253, -42.467)
  point P166 (26.265, -43.7071)
  point P167 (25.9463, -44.2207)
  point P168 (25.6977, -44.6448)
  point P169 (25.5601, -44.9191)
  point P170 (25.4213, -45.1259)
  point P171 (25.3358, -45.2768)
  point P172 (25.3438, -45.4679)
  point P173 (25.3384, -45.6277)
  point P174 (25.3834, -45.7748)
  point P175 (25.4739, -45.8543)
  point P176 (25.829, -46.276)
  point P177 (26.1163, -46.6339)
  point P178 (26.361, -46.9851)
  point P179 (26.5639, -47.1679)
  point P180 (26.7607, -47.3986)
  point P181 (26.9498, -47.5547)
  point P182 (27.2153, -47.591)
  point P183 (27.681, -47.5666)
  point P184 (28.1725, -47.5635)
  point P185 (28.5519, -47.6906)
  point P186 (28.9926, -48.1263)
  point P187 (29.218, -48.3489)
  point P188 (29.5352, -48.5784)
  point P189 (29.92, -48.8657)
  point P190 (30.3438, -49.0938)
  point P191 (31.3356, -49.6055)
  point P192 (32.4397, -50.1554)
  point P193 (33.8492, -50.6659)
  point P194 (34.4831, -50.8187)
  point P195 (34.8108, -50.9516)
  point P196 (35.4816, -51.2518)
  point P197 (36.098, -51.543)
  point P198 (36.4606, -51.7)
  point P199 (36.6489, -51.7611)
  constraints: 218 symmetric about line, 68 end point, 44 point on circle, 24 centre point, 11 horizontal, 8 vertical, 5 point on line, 1 coincident, 1 midpoint, 1 perpendicular, 261 other
extrude "Extrusion1" add sketch "Sketch1" along normal blind 1.5 contours A0 | L4 L5 S0 L6 A2 L7 A3 L8 A4 L9 S1 A5 S2 L42 L43 L44 L194 L45 | L194 L44 L85 L84 S5 A9 S4 L51 A8 L50 A7 L49 A6 L48 S3 L47 L46 L45 | L303 S17 S18 S19 S20 S21 L302 L194 A21 A20 A19 A17 A18 L195 L196 S9 S10 L287 L286 S11 L300 | L194 L193 S8 L179 L180 S7 S6 L89 L88 A16 A15 A14 A13 A12 A11 A10 L87 S16 S15 S14 S13 S12 L301
sketch "Sketch2" plane through (0, 1.5, 0) normal (0, 1, 0) x (1, 0, 0)
  circle A0 centre (-38.1001, 38.1001) radius 21.8573 projected
  point P0 (0, 0)
extrude "Extrusion2" add sketch "Sketch2" along normal blind 4.85
body "Solid1"
